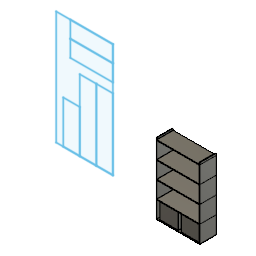
Book Shelves v1 (Autodesk Fusion 360 design; units mm, degrees)
Autodesk Fusion 360 part; units mm, degrees
sketch "Sketch1" plane through (0, 0, 0) normal (0, 1, 0) x (1, 0, 0)
  line L0 (0, 0) -> (36, 0)
  line L1 (36, 0) -> (36, -14)
  line L2 (36, -14) -> (0, -14)
  line L3 (0, -14) -> (0, 0)
  dimension "d1" = 14
  dimension "d2" = 36
  constraint horizontal L0
  constraint vertical L1
  constraint horizontal L2
  constraint vertical L3
  constraint coincident L0.start L3.end
  measures "d1" distance of L0.start L2.end
  measures "d2" distance of L0.start L0.end
extrude "Extrude1" add sketch "Sketch1" along normal blind 0.5 makes body 1
sketch "Sketch2" plane through (0, 0.5, 0) normal (0, 1, 0) x (-1, 0, 0)
  line L0 (0, 14) -> (-36, 14)
  line L1 (-36, 14) -> (-36, 0)
  line L2 (-36, 0) -> (0, 0)
  line L3 (0, 0) -> (0, 14)
  line L4 (0, 0) -> (-15.5, 0)
  line L5 (-15.5, 0) -> (-15.5, 13.25)
  line L6 (-15.5, 13.25) -> (0, 13.25)
  line L7 (0, 13.25) -> (0, 0)
  dimension "d5" = 15.5
  dimension "d6" = 13.25
  constraint horizontal L4
  constraint vertical L5
  constraint horizontal L6
  constraint vertical L7
  constraint coincident L2.end L3.start
  measures "d5" distance of L2.end L4.end
  measures "d6" distance of L2.end L6.end
extrude "Extrude2" add sketch "Sketch2" along normal blind 13.5 separate body contours L2 L3 L4 L5 L6 L7 makes body 2
copy_body "CopyPasteBodies1" bodies 1 makes body 3
move_body "Move1" bodies 3 to x (1, 0, 0) y (0, 1, 0) z (0, 0, 1) at (0, 14.5, 0)
copy_body "CopyPasteBodies2" bodies 3 makes body 4
move_body "Move2" bodies 4 to x (1, 0, 0) y (0, 1, 0) z (0, 0, 1) at (0, 14.5, 0)
copy_body "CopyPasteBodies3" bodies 4 makes body 5
move_body "Move3" bodies 5 to x (1, 0, 0) y (0, 1, 0) z (0, 0, 1) at (0, 14.5, 0)
copy_body "CopyPasteBodies4" bodies 5 makes body 6
move_body "Move4" bodies 6 to x (1, 0, 0) y (0, 1, 0) z (0, 0, 1) at (0, 14.5, 0)
extrude "Extrude3" cut 1 faces at (12, 58.5, 4.6667) along direction (0, -1, 0) blind 2 on bodies 6 bodies 6
sketch "Sketch3" plane through (0, 44, 0) normal (0, 1, 0) x (-1, 0, 0)
  line L0 (0, 14) -> (-36, 14)
  line L1 (-36, 14) -> (-36, 0)
  line L2 (-36, 0) -> (0, 0)
  line L3 (0, 0) -> (0, 14)
  line L4 (0, 0) -> (0.5, 0)
  line L5 (0.5, 0) -> (0.5, 14)
  line L6 (0.5, 14) -> (0, 14)
  line L7 (0, 14) -> (0, 0)
  line L8 (-36, 0) -> (-36.5, 0)
  line L9 (-36.5, 0) -> (-36.5, 14)
  line L10 (-36.5, 14) -> (-36, 14)
  line L11 (-36, 14) -> (-36, 0)
  dimension "d11" = 0.5
  dimension "d12" = 0.5
  constraint horizontal L4
  constraint vertical L5
  constraint horizontal L6
  constraint vertical L7
  constraint coincident L2.end L3.start
  constraint horizontal L8
  constraint vertical L9
  constraint horizontal L10
  constraint vertical L11
  constraint coincident L1.end L2.start
  measures "d11" distance of L2.end L4.end
  measures "d12" distance of L1.end L8.end
extrude "Extrude4" add sketch "Sketch3" against normal blind 44 separate body contours L3 L4 L5 L6 L7 | L1 L8 L9 L10 L11 makes body 7 at (36.5, 29.3333, 4.6667) makes body 8 at (-0.5, 29.3333, 4.6667)
copy_body "CopyPasteBodies5" bodies 2 makes body 9
move_body "Move5" bodies 9 to x (1, 0, 0) y (0, 1, 0) z (0, 0, 1) at (20, 0, 0)
move_body "Move6" bodies 2 to x (1, 0, 0) y (0, 1, 0) z (0, 0, 1) at (2, 0, 0)
copy_body "CopyPasteBodies6" bodies 5 makes body 10
move_body "Move7" bodies 10 to x (1, 0, 0) y (0, 1, 0) z (0, 0, 1) at (0, 14.5, 0)
extrude "Extrude5" add 2 faces at (36.3333, 44, 9.3333) (-0.3333, 44, 9.3333) along direction (0, 1, 0) blind 16 on bodies 7 8 bodies 7 5 6 8
sketch "Sketch4" plane through (0, 0, 0) normal (0, 0, 1) x (1, 0, 0)
  line L0 (-51, 0) -> (-99, 0)
  line L1 (-99, 0) -> (-99, 96)
  line L2 (-99, 96) -> (-51, 96)
  line L3 (-51, 96) -> (-51, 0)
  line L4 (-51, 0) -> (-65, 0)
  line L5 (-65, 0) -> (-65, 60)
  line L6 (-65, 60) -> (-51, 60)
  line L7 (-51, 60) -> (-51, 0)
  line L8 (-65, 60) -> (-79, 60)
  line L9 (-79, 60) -> (-79, 0)
  line L10 (-79, 0) -> (-65, 0)
  line L11 (-65, 0) -> (-65, 60)
  line L12 (-51, 96) -> (-87, 96)
  line L13 (-87, 96) -> (-87, 82)
  line L14 (-87, 82) -> (-51, 82)
  line L15 (-51, 82) -> (-51, 96)
  line L16 (-51, 82) -> (-87, 82)
  line L17 (-87, 82) -> (-87, 68)
  line L18 (-87, 68) -> (-51, 68)
  line L19 (-51, 68) -> (-51, 82)
  line L20 (-79, 0) -> (-93, 0)
  line L21 (-93, 0) -> (-93, 36)
  line L22 (-93, 36) -> (-79, 36)
  line L23 (-79, 36) -> (-79, 0)
  dimension "d17" = 96
  dimension "d18" = 48
  dimension "d19" = 60
  dimension "d20" = 14
  dimension "d21" = 14
  dimension "d22" = 36
  dimension "d23" = 14
  dimension "d24" = 14
  dimension "d25" = 14
  dimension "d26" = 36
  constraint horizontal L0
  constraint vertical L1
  constraint horizontal L2
  constraint vertical L3
  constraint horizontal L4
  constraint vertical L5
  constraint horizontal L6
  constraint vertical L7
  constraint horizontal L8
  constraint vertical L9
  constraint horizontal L10
  constraint vertical L11
  constraint horizontal L12
  constraint vertical L13
  constraint horizontal L14
  constraint vertical L15
  constraint horizontal L16
  constraint vertical L17
  constraint horizontal L18
  constraint vertical L19
  constraint horizontal L20
  constraint vertical L21
  constraint horizontal L22
  constraint vertical L23
  measures "d17" distance of L0.start L2.end
  measures "d18" distance of L0.start L0.end
  measures "d19" distance of L0.start L6.end
  measures "d20" distance of L0.start L4.end
  measures "d21" distance of L5.end L8.end
  measures "d22" distance of L2.end L12.end
  measures "d23" distance of L2.end L14.end
  measures "d24" distance of L14.end L18.end
  measures "d25" distance of L9.end L20.end
  measures "d26" distance of L9.end L22.end
